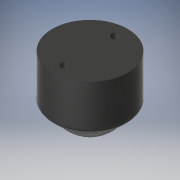
# Autodesk Inventor part: 0.75in Ball Caster (Pololu)
Saved by Autodesk Inventor 2019.4 (Build 234330000, 330)
## iProperties
Created: 2014-04-22
Part Number: 0.75in Ball Caster (Pololu)
Material: Stainless Steel
Document SubType Name: Modeling
Designer: Mike Angus
Density: 8 g/cm^3
Appearance: Semi-Polished
Sending System: SolidWorks 2013
Last Author: Slydog
Last Saved: 2014-06-05
Author: Mike Angus
Autodesk Inventor part; units mm, degrees
ref_plane "YZ Plane" through (0, 0, 0) normal (1, 0, 0) x (0, 1, 0)
ref_plane "XY Plane" through (0, 0, 0) normal (0, 0, 1) x (1, 0, 0)
sketch "Sketch1" plane through (0, 0, 0) normal (0, 0, 1) x (1, 0, 0)
  line L0 (0, 9.525) -> (0, -9.525)
  arc A0 (0, -9.525) -> (0, 9.525) centre (0, 0) ccw
  dimension "d0" = 19.05
  constraints: 2 coincident, 2 end point, 2 point on circle, 1 centre point, 1 midpoint, 1 vertical
  measures "d0" distance of L0.start L0.end
revolve "Revolution1" add sketch "Sketch1" angle 360 about axis through (0, 9.525, 0) along (0, -1, 0)
ref_plane "Work Plane1" through (0, 9.525, 0) normal (0, 1, 0) x (-1, 0, 0)
ref_plane "Work Plane3" through (0, 11.175, 0) normal (0, 1, 0) x (-1, 0, 0)
ref_plane "Work Plane2" through (0, -9.525, 0) normal (0, 1, 0) x (-1, 0, 0)
sketch "Sketch2" plane through (0, 11.175, 0) normal (0, 1, 0) x (-1, 0, 0)
  circle A0 centre (0, 0) radius 11.5
  dimension "d2" = 23
  constraints: 1 centre point, 1 coincident
  measures "d2" diameter of A0
extrude "Extrusion1" add sketch "Sketch2" against normal blind 14.6 separate body
chamfer "Chamfer1" distance 1.5 angle 45 1 edges at (11.5, -3.425, 0)
fillet "Fillet1" radius 1 2 edges at (10, -3.425, 0) (11.5, -1.925, 0)
sketch "Sketch3" plane through (0, 11.175, 0) normal (0, 1, 0) x (1, 0, 0)
  line L0 (0, -7.7) -> (0, 7.7) construction
  circle A0 centre (0, -7.7) radius 1.27
  circle A1 centre (0, 7.7) radius 1.27
  point P0 (0, 0)
  point P1 (0, 0)
  dimension "d11" = 15.4
  dimension "d12" = 2.54
  dimension "d13" = 2.54
  constraints: 3 coincident, 2 centre point, 2 end point, 1 midpoint, 1 vertical
  measures "d11" distance of L0.start L0.end
  measures "d12" diameter of A0
  measures "d13" diameter of A1
extrude "Extrusion2" cut sketch "Sketch3" against normal blind 14.6 bodies 2
body "Solid3"
body "Solid4"
